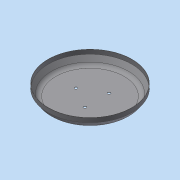
# Autodesk Inventor part: Saucer
Saved by Autodesk Inventor 2015 SP1 (Build 190203100, 203)
## iProperties
Created: 2015-01-29
Part Number: Saucer
Material: Generic
Document SubType Name: Modeling
Designer: Jostein
Density: 1 g/cm^3
Appearance: Default
Author: Jostein
Autodesk Inventor part; units mm, degrees
ref_plane "YZ Plane" through (0, 0, 0) normal (1, 0, 0) x (0, 1, 0)
ref_plane "XZ Plane" through (0, 0, 0) normal (0, 1, 0) x (-1, 0, 0)
ref_plane "XY Plane" through (0, 0, 0) normal (0, 0, 1) x (1, 0, 0)
sketch "Sketch2" plane through (0, 0, 0) normal (0, 1, 0) x (-1, 0, 0)
  line L0 (0, 0) -> (-610.4174, 0)
  line L1 (-692.3326, 42.6424) -> (-750, 125)
  line L2 (-750, 200) -> (0, 200)
  line L3 (0, 200) -> (0, 0)
  arc A0 (-692.3326, 42.6424) -> (-610.4174, 0) centre (-610.4174, 100) ccw
  line L4 (-750, 200) -> (-750, 125)
  dimension "d0" = 100
  dimension "d1" = 200
  dimension "d2" = 750
  dimension "d3" = 125
  dimension "d4" = 75
  constraints: 10 end point, 2 perpendicular, 2 point on circle, 2 tangent, 1 centre point, 1 horizontal, 1 parallel
  measures "d0" radius of A0
  measures "d1" distance of L2.end L0.start
  measures "d2" distance of L2.start L2.end
  measures "d3" angle of L0 L1
  measures "d4" distance of L2.start L1.end
revolve "Revolution1" add sketch "Sketch2" angle 360 about axis through (0, 0, 200) along (0, 0, -1)
shell "Shell1" thickness 5 removed faces 1 at (-44.9023, -186.6904, 200)
sketch "Sketch4" plane through (0, 0, 0) normal (0, 0, -1) x (-1, 0, 0)
  line L0 (1050, 0) -> (-1050, 0) construction
  line L1 (0, -1050) -> (0, 1050) construction
  circle A0 centre (-125, -216.5064) radius 25
  line L2 (-125, -216.5064) -> (0, 0) construction
  circle A1 centre (250, 0) radius 25
  circle A2 centre (-125, 216.5064) radius 25
  dimension "d8" = 50
  dimension "d9" = 60
  dimension "d10" = 250
  dimension "d13" = 360
  constraints: 3 centre point, 2 end point, 7 other
  measures "d8" diameter of A0
  measures "d9" angle of L0 L2
  measures "d10" distance of L2.start L2.end
extrude "Extrusion1" cut sketch "Sketch4" against normal through all
body "Solid1"
